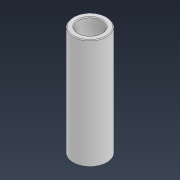
# Autodesk Inventor part: Sworzeń tłoka
Saved by Autodesk Inventor 2022 (Build 260153000, 153)
## iProperties
Created: 2023-04-17
Part Number: Sworzeń tłoka
Material: Generic
Document SubType Name: Modeling
Designer: wikto
Density: 1 g/cm^3
Appearance: Default
Author: wikto
Autodesk Inventor part; units mm, degrees
ref_plane "YZ Plane" through (0, 0, 0) normal (1, 0, 0) x (0, 1, 0)
ref_plane "XZ Plane" through (0, 0, 0) normal (0, 1, 0) x (-1, 0, 0)
ref_plane "XY Plane" through (0, 0, 0) normal (0, 0, 1) x (1, 0, 0)
sketch "Sketch1" plane through (0, 0, 0) normal (0, 1, 0) x (-1, 0, 0)
  circle A0 centre (0, 0) radius 11
  circle A1 centre (0, 0) radius 7.5
  dimension "d0" = 22
  dimension "d1" = 15
  constraints: 2 centre point, 2 coincident
  measures "d0" diameter of A0
  measures "d1" diameter of A1
extrude "Extrusion1" add sketch "Sketch1" along normal blind 72
chamfer "Chamfer1" distance 0.5 angle 45 4 edges at (7.5, 72, 0) (11, 72, 0) (11, 0, 0) (7.5, 0, 0)
body "Solid1"
